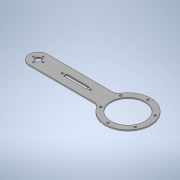
# Autodesk Inventor part: ForeArm_outside_frame_
Saved by Autodesk Inventor 2020.4 (Build 244396000, 396)
## iProperties
Created: 2022-01-10
Part Number: ForeArm_outside_frame_
Material: GFRP
Document SubType Name: Modeling
Designer: Masato Kubotera
Density: 1.75 g/cm^3
Appearance: 滑らか - 標準の灰色
Author: Masato Kubotera
Autodesk Inventor part; units mm, degrees
ref_plane "YZ Plane" through (0, 0, 0) normal (1, 0, 0) x (0, 1, 0)
ref_plane "XZ Plane" through (0, 0, 0) normal (0, 1, 0) x (-1, 0, 0)
ref_plane "XY Plane" through (0, 0, 0) normal (0, 0, 1) x (1, 0, 0)
sketch "スケッチ1" plane through (0, 0, 0) normal (0, 1, 0) x (-1, 0, 0)
  circle A0 centre (0, 0) radius 5.05
  line L0 (0, 8.5) -> (0, -8.5) construction
  circle A1 centre (0, 8.5) radius 1.35
  circle A2 centre (-8.5, 0) radius 1.35
  circle A3 centre (0, -8.5) radius 1.35
  circle A4 centre (8.5, 0) radius 1.35
  circle A5 centre (0, -158.8519) radius 16 construction
  line L1 (0, 0) -> (0, -158.8519) construction
  arc A6 (-16, -121.8654) -> (16, -121.8654) centre (0, -158.8519) ccw
  circle A7 centre (0, 8.5) radius 2.4 construction
  line L2 (-16, 31) -> (16, 31) construction
  line L3 (16, 31) -> (16, -12) construction
  line L4 (16, -12) -> (-16, -12) construction
  line L5 (-16, -12) -> (-16, 31) construction
  line L6 (-16, 31) -> (16, -12) construction
  line L7 (16, 31) -> (-16, -12) construction
  arc A8 (-16, 0) -> (-10.583, -12) centre (0, 0) ccw construction
  arc A9 (10.583, -12) -> (16, 0) centre (0, 0) ccw construction
  line L8 (-16, -121.8654) -> (-16, 0)
  line L9 (16, -121.8654) -> (16, 0)
  circle A10 centre (0, -92.5) radius 1.6
  line L10 (0, -158.8519) -> (-20.1494, -123.952) construction
  circle A11 centre (-17.6494, -128.2822) radius 5 construction
  circle A12 centre (-17.6494, -128.2822) radius 2
  circle A13 centre (-35.2989, -158.8519) radius 2
  circle A14 centre (-17.6494, -189.4216) radius 2
  circle A15 centre (17.6494, -189.4216) radius 2
  circle A16 centre (35.2989, -158.8519) radius 2
  circle A17 centre (17.6494, -128.2822) radius 2
  circle A18 centre (0, -158.8519) radius 58.8961 construction
  line L11 (30.6064, -21.0119) -> (2.8936, -37.0119) construction
  line L12 (2.8936, -37.0119) -> (-18.6064, 0.2272) construction
  line L13 (-18.6064, 0.2272) -> (9.1064, 16.2272) construction
  line L14 (9.1064, 16.2272) -> (30.6064, -21.0119) construction
  line L15 (30.6064, -21.0119) -> (-18.6064, 0.2272) construction
  line L16 (2.8936, -37.0119) -> (9.1064, 16.2272) construction
  line L17 (16.75, -29.0119) -> (-4.75, 8.2272) construction
  circle A19 centre (0, -42.5) radius 1.6
  line L18 (-2.5, -47.5) -> (2.5, -47.5) construction
  line L19 (2.5, -47.5) -> (2.5, -57.5) construction
  line L20 (2.5, -57.5) -> (-2.5, -57.5) construction
  line L21 (-2.5, -57.5) -> (-2.5, -47.5) construction
  line L22 (-2.5, -47.5) -> (2.5, -57.5) construction
  line L23 (2.5, -47.5) -> (-2.5, -57.5) construction
  line L24 (-2.5, -52.5) -> (2.5, -52.5) construction
  circle A20 centre (0, -62.5) radius 1.6
  line L25 (2.8936, -37.0119) -> (54.9285, -127.1389) construction
  line L26 (0, -158.8519) -> (54.9285, -127.1389) construction
  line L27 (-2.5, -47.5) -> (2.5, -47.5) construction
  line L28 (2.5, -47.5) -> (2.5, -87.5) construction
  line L29 (2.5, -87.5) -> (-2.5, -87.5) construction
  line L30 (-2.5, -87.5) -> (-2.5, -47.5) construction
  line L31 (-2.5, -47.5) -> (2.5, -87.5) construction
  line L32 (2.5, -47.5) -> (-2.5, -87.5) construction
  line L33 (-2.55, -47.45) -> (2.55, -47.45)
  line L34 (2.55, -47.45) -> (2.55, -87.55)
  line L35 (2.55, -87.55) -> (-2.55, -87.55)
  line L36 (-2.55, -87.55) -> (-2.55, -47.45)
  line L37 (-2.55, -47.45) -> (2.55, -87.55) construction
  line L38 (2.55, -47.45) -> (-2.55, -87.55) construction
  arc A21 (-1.0651, -47.45) -> (-2.55, -48.9349) centre (-1.8075, -48.1925) ccw
  arc A22 (2.55, -48.9349) -> (1.0651, -47.45) centre (1.8075, -48.1925) ccw
  line L39 (-2.5, -67.5) -> (2.5, -67.5) construction
  arc A23 (-2.55, -86.0651) -> (-1.0651, -87.55) centre (-1.8075, -86.8075) ccw
  arc A24 (1.0651, -87.55) -> (2.55, -86.0651) centre (1.8075, -86.8075) ccw
  arc A25 (16, 0) -> (-16, 0) centre (0, 0) ccw
  circle A26 centre (0, -158.8519) radius 30.2989
  point P0 (0, 9.5)
  point P1 (0, 9.5)
  point P2 (6, -10.3923)
  point P3 (0, -52.5)
  point P4 (0, -67.5)
  point P5 (1.0651, -87.55)
  point P6 (-1.0651, -87.55)
  point P7 (-2.55, -86.0651)
  point P8 (2.55, -48.9349)
  point P9 (2.55, -86.0651)
  dimension "d0" = 10.1
  dimension "d1" = 17
  dimension "d2" = 2.7
  dimension "d5" = 360
  dimension "d7" = 32
  dimension "d8" = 158.8519
  dimension "d9" = 80.5978
  dimension "d10" = 4.8
  dimension "d11" = 32
  dimension "d12" = 43
  dimension "d14" = 9.5
  dimension "d17" = 3.2
  dimension "d23" = 32
  dimension "d24" = 30
  dimension "d25" = 10
  dimension "d26" = 4
  dimension "d29" = 360
  dimension "d32" = 117.7922
  dimension "d33" = 32
  dimension "d34" = 43
  dimension "d36" = 9.5
  dimension "d37" = 150
  dimension "d38" = 3.2
  dimension "d40" = 5
  dimension "d41" = 10
  dimension "d42" = 50
  dimension "d43" = 20
  dimension "d44" = 42.5
  dimension "d45" = 40
  dimension "d46" = 1.05
  dimension "d47" = 0.05
  dimension "d48" = 0.05
  dimension "d49" = 16
  constraints: 81 end point, 27 centre point, 18 midpoint, 18 point on circle, 14 symmetric about line, 11 point on line, 10 coincident, 10 parallel, 6 perpendicular, 4 horizontal, 4 tangent, 3 collinear, 2 vertical, 27 other
  measures "d0" diameter of A0
  measures "d1" distance of L0.start L0.end
  measures "d2" diameter of A1
  measures "d7" diameter of A5
  measures "d8" distance of L1.end point (0, 0)
  measures "d9" diameter of A6
  measures "d10" diameter of A7
  measures "d11" distance of L3.end L4.end
  measures "d12" distance of L2.end L3.end
  measures "d14" distance of point (0, 0) point (0, 9.5)
  measures "d17" diameter of A10
  measures "d23" distance of L9.start L8.start
  measures "d24" angle of L10 L1
  measures "d25" diameter of A11
  measures "d26" diameter of A12
  measures "d32" diameter of A18
  measures "d33" distance of L12.end L13.end
  measures "d34" distance of L11.end L12.end
  measures "d36" distance of L17.end point (0, 0)
  measures "d37" angle of L1 L12
  measures "d38" diameter of A19
  measures "d40" distance of L19.end L20.end
  measures "d41" distance of L18.end L19.end
  measures "d42" distance of A10.centre A19.centre
  measures "d43" distance of A20.centre A19.centre
  measures "d44" distance of A19.centre point (0, 0)
  measures "d45" distance of L27.end L28.end
  measures "d46" radius of A21
  measures "d47" distance between parallel lines of L33 L27
  measures "d48" distance between parallel lines of L36 L30
  measures "d49" radius of A25
extrude "押し出し1" add sketch "スケッチ1" along normal blind 2 contours L8 A25 L9 A6
fillet "フィレット1" radius 10 2 edges at (16, 1, -121.8654) (-16, 1, -121.8654)
equation "\"d36\" = d14"
